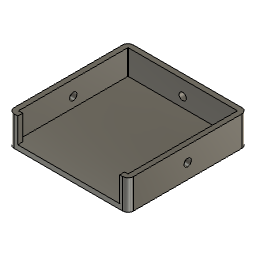
Mad Eye v2 (Autodesk Fusion 360 design; units mm, degrees)
Autodesk Fusion 360 part; units mm, degrees
box "BoxPrimitive1" add length 48 width 48 height 12 placed x (0, 1, 0) y (-1, 0, 0) z (0, 0, 1) at (45.6849, 0, 0)
fillet "Fillet1" radius 2.19 4 edges at (45.6849, 0, 6) (45.6849, 48, 6) (-2.3151, 48, 6) (-2.3151, 0, 6)
shell "Shell1" thickness 2 removed faces 1 at (14.4149, 17.46, 12)
box "BoxPrimitive2" cut length 24.625 width 40.955 height 12.783 placed x (0, -1, 0) y (1, 0, 0) z (0, 0, 1) at (1.3626, 16.0218, 2)
hole "Hole1" at (45.6849, 24, 6) direction (-1, 0, 0) diameter 2.95 depth 10 tip angle 118
hole "Hole2" at (21.6849, 48, 6) direction (0, -1, 0) diameter 2.95 depth 10 tip angle 118
hole "Hole3" at (-2.3151, 24, 6) direction (1, 0, 0) diameter 2.95 depth 10 tip angle 118
